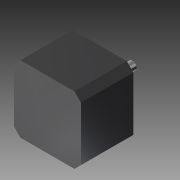
# Autodesk Inventor part: stepper_short
Saved by Autodesk Inventor 2013 (Build 170138000, 138)
## iProperties
Created: 2013-07-22
Part Number: stepper_short
Material: Generic
Document SubType Name: Modeling
Designer: dkboone
Density: 1 g/cm^3
Author: dkboone
Autodesk Inventor part; units mm, degrees
ref_plane "YZ Plane" through (0, 0, 0) normal (1, 0, 0) x (0, 1, 0)
ref_plane "XZ Plane" through (0, 0, 0) normal (0, 1, 0) x (-1, 0, 0)
ref_plane "XY Plane" through (0, 0, 0) normal (0, 0, 1) x (1, 0, 0)
sketch "Sketch1" plane through (0, 0, 0) normal (0, 1, 0) x (-1, 0, 0)
  line L0 (16.5, -20.5) -> (-16.5, -20.5)
  line L1 (-20.5, -16.5) -> (-20.5, 16.5)
  line L2 (-16.5, 20.5) -> (16.5, 20.5)
  line L3 (20.5, 16.5) -> (20.5, -16.5)
  line L4 (20.5, -16.5) -> (16.5, -20.5)
  line L5 (-16.5, -20.5) -> (-20.5, -16.5)
  line L6 (-20.5, 16.5) -> (-16.5, 20.5)
  line L7 (16.5, 20.5) -> (20.5, 16.5)
  point P0 (0, 0)
  point P1 (20.5, -20.5)
  point P2 (-20.5, 20.5)
  point P3 (-20.5, -20.5)
  point P4 (20.5, 20.5)
  dimension "d0" = 41
  dimension "d2" = 41
  dimension "d3" = 20.5
  dimension "d4" = 20.5
  dimension "d5" = 4
  dimension "d6" = 4
  dimension "d7" = 4
  dimension "d8" = 4
  dimension "d9" = 4
  dimension "d10" = 4
  dimension "d11" = 4
  dimension "d12" = 4
  constraints: 16 end point, 8 point on line, 2 parallel, 1 horizontal, 1 perpendicular
  measures "d0" distance of point (20.5, -20.5) point (-20.5, -20.5)
  measures "d2" distance of point (-20.5, -20.5) point (-20.5, 20.5)
  measures "d3" distance from line of point (0, 0) L0
  measures "d4" distance from line of point (0, 0) L3
  measures "d5" distance of L3.end point (20.5, -20.5)
  measures "d6" distance of L0.start point (20.5, -20.5)
  measures "d7" distance of L0.end point (-20.5, -20.5)
  measures "d8" distance of L1.start point (-20.5, -20.5)
  measures "d9" distance of L1.end point (-20.5, 20.5)
  measures "d10" distance of L2.start point (-20.5, 20.5)
  measures "d11" distance of L2.end point (20.5, 20.5)
  measures "d12" distance of L3.start point (20.5, 20.5)
extrude "Extrusion1" add sketch "Sketch1" against normal blind 32
sketch "Sketch4" plane through (0, 0, 0) normal (0, 1, 0) x (-1, 0, 0)
  circle A0 centre (0, 0) radius 11.5
  circle A1 centre (0, 0) radius 4.75
  dimension "d24" = 23
  dimension "d26" = 9.5
  constraints: 2 centre point, 2 coincident
  measures "d24" diameter of A0
  measures "d26" diameter of A1
extrude "Extrusion4" add sketch "Sketch4" along normal blind 2
sketch "Sketch5" plane through (0, 0, 0) normal (0, 1, 0) x (-1, 0, 0)
  circle A0 centre (0, 0) radius 2.5
  dimension "d29" = 5
  constraints: 1 centre point, 1 coincident
  measures "d29" diameter of A0
extrude "Extrusion5" add sketch "Sketch5" along normal blind 20
sketch "Sketch6" plane through (0, 0, 0) normal (0, 1, 0) x (1, 0, 0)
  line L0 (-20.5, -16.5) -> (-20.5, 16.5) projected
  line L1 (-16.5, 20.5) -> (16.5, 20.5) projected
  circle A0 centre (0, 0) radius 11.5 projected
  point P0 (-15.5, 15.5)
  point P1 (-15.5, -15.5)
  point P2 (15.5, 15.5)
  point P3 (15.5, -15.5)
  dimension "d33" = 15.5
  dimension "d34" = 15.5
  dimension "d37" = 31
  dimension "d40" = 31
  constraints: 1 horizontal, 1 vertical, 3 other
  measures "d33" horizontal distance of point (-15.5, 15.5) A0.centre
  measures "d34" horizontal distance of A0.centre point (-15.5, 15.5)
  measures "d37" distance of point (-15.5, 15.5) point (-15.5, -15.5)
  measures "d40" distance of point (-15.5, 15.5) point (15.5, 15.5)
hole "Hole1" at (-15.5, 0, -15.5) at (-15.5, 0, 15.5) at (15.5, 0, -15.5) at (15.5, 0, 15.5) direction (0, -1, 0) diameter 2.5 depth 8 tip angle 118
thread "Thread1" size "M2.5x0.45" class "6H" standard "ANSI Metric M Profile" full length
thread "Thread2" size "M2.5x0.45" class "6H" standard "ANSI Metric M Profile" full length
thread "Thread3" size "M2.5x0.45" class "6H" standard "ANSI Metric M Profile" full length
thread "Thread4" size "M2.5x0.45" class "6H" standard "ANSI Metric M Profile" full length
equation "\"d3\" = 0.5 * d2"
equation "\"d4\" = 0.5 * d0"
equation "\"d6\" = d5"
equation "\"d7\" = d5"
equation "\"d8\" = d7"
equation "\"d9\" = d5"
equation "\"d10\" = d9"
equation "\"d11\" = d5"
equation "\"d12\" = d11"
equation "\"d33\" = 0.5 * d37"
equation "\"d34\" = d33"
body "Solid1"
